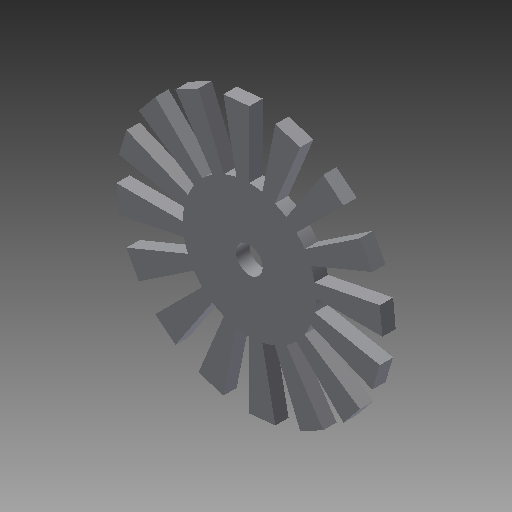
# Autodesk Inventor part: encoder
Saved by Autodesk Inventor 2017 (Build 210142000, 142)
## iProperties
Created: 2016-09-12
Part Number: encoder
Material: Generic
Document SubType Name: Modeling
Designer: Paulo Loma
Density: 1 g/cm^3
Appearance: Default
Author: Paulo Loma
Autodesk Inventor part; units mm, degrees
ref_plane "YZ Plane" through (0, 0, 0) normal (1, 0, 0) x (0, 1, 0)
ref_plane "XZ Plane" through (0, 0, 0) normal (0, 1, 0) x (-1, 0, 0)
ref_plane "XY Plane" through (0, 0, 0) normal (0, 0, 1) x (1, 0, 0)
sketch "Sketch1" plane through (0, 0, 0) normal (0, 0, 1) x (1, 0, 0)
  circle A0 centre (0, 0) radius 1
  circle A1 centre (0, 0) radius 5
  line L0 (1.9509, 9.8079) -> (3.8268, 9.2388)
  line L1 (5.5557, 8.3147) -> (7.0711, 7.0711)
  line L2 (8.3147, 5.5557) -> (9.2388, 3.8268)
  line L3 (9.8079, 1.9509) -> (10, 0)
  line L4 (9.8079, -1.9509) -> (9.2388, -3.8268)
  line L5 (8.3147, -5.5557) -> (7.0711, -7.0711)
  line L6 (5.5557, -8.3147) -> (3.8268, -9.2388)
  line L7 (1.9509, -9.8079) -> (0, -10)
  line L8 (-1.9509, -9.8079) -> (-3.8268, -9.2388)
  line L9 (-5.5557, -8.3147) -> (-7.0711, -7.0711)
  line L10 (-8.3147, -5.5557) -> (-9.2388, -3.8268)
  line L11 (-9.8079, -1.9509) -> (-10, 0)
  line L12 (-9.8079, 1.9509) -> (-9.2388, 3.8268)
  line L13 (-8.3147, 5.5557) -> (-7.0711, 7.0711)
  line L14 (-5.5557, 8.3147) -> (-3.8268, 9.2388)
  line L15 (-1.9509, 9.8079) -> (0, 10)
  line L16 (-3.8268, 9.2388) -> (-1.9134, 4.6194)
  line L17 (-5.5557, 8.3147) -> (-2.7779, 4.1573)
  line L18 (-9.2388, -3.8268) -> (-4.6194, -1.9134)
  line L19 (-8.3147, -5.5557) -> (-4.1573, -2.7779)
  line L20 (-7.0711, -7.0711) -> (-3.5355, -3.5355)
  line L21 (-5.5557, -8.3147) -> (-2.7779, -4.1573)
  line L22 (-1.9509, -9.8079) -> (-0.9755, -4.9039)
  line L23 (-3.8268, -9.2388) -> (-1.9134, -4.6194)
  line L24 (0, -5) -> (0, -10)
  line L25 (0.9755, -4.9039) -> (1.9509, -9.8079)
  line L26 (-0.3827, 0.9239) -> (0.3827, -0.9239)
  line L27 (1.9134, -4.6194) -> (3.8268, -9.2388)
  line L28 (-0.5556, 0.8315) -> (0.5556, -0.8315)
  line L29 (2.7779, -4.1573) -> (5.5557, -8.3147)
  line L30 (3.5355, -3.5355) -> (7.0711, -7.0711)
  line L31 (4.1573, -2.7779) -> (8.3147, -5.5557)
  line L32 (4.6194, -1.9134) -> (9.2388, -3.8268)
  line L33 (4.9039, -0.9755) -> (9.8079, -1.9509)
  line L34 (5, 0) -> (10, 0)
  line L35 (4.9039, 0.9755) -> (9.8079, 1.9509)
  line L36 (-0.9239, -0.3827) -> (0.9239, 0.3827)
  line L37 (4.6194, 1.9134) -> (9.2388, 3.8268)
  line L38 (-0.8315, -0.5556) -> (0.8315, 0.5556)
  line L39 (4.1573, 2.7779) -> (8.3147, 5.5557)
  line L40 (-0.7071, -0.7071) -> (0.7071, 0.7071)
  line L41 (3.5355, 3.5355) -> (7.0711, 7.0711)
  line L42 (-0.5556, -0.8315) -> (0.5556, 0.8315)
  line L43 (2.7779, 4.1573) -> (5.5557, 8.3147)
  line L44 (-0.3827, -0.9239) -> (0.3827, 0.9239)
  line L45 (1.9134, 4.6194) -> (3.8268, 9.2388)
  line L46 (-0.1951, -0.9808) -> (0.1951, 0.9808)
  line L47 (0.9755, 4.9039) -> (1.9509, 9.8079)
  line L48 (0, 10) -> (0, 5)
  line L49 (0, 1) -> (0, -1)
  line L50 (-1.9509, 9.8079) -> (-0.9755, 4.9039)
  line L51 (-0.1951, 0.9808) -> (0.1951, -0.9808)
  line L52 (-7.0711, 7.0711) -> (-3.5355, 3.5355)
  line L53 (-0.7071, 0.7071) -> (0.7071, -0.7071)
  line L54 (-8.3147, 5.5557) -> (-4.1573, 2.7779)
  line L55 (-0.8315, 0.5556) -> (0.8315, -0.5556)
  line L56 (-9.2388, 3.8268) -> (-4.6194, 1.9134)
  line L57 (-0.9239, 0.3827) -> (0.9239, -0.3827)
  line L58 (-0.9808, 0.1951) -> (0.9808, -0.1951)
  line L59 (-10, 0) -> (-5, 0)
  line L60 (-1, 0) -> (1, 0)
  line L61 (-9.8079, -1.9509) -> (-4.9039, -0.9755)
  line L62 (-0.9808, -0.1951) -> (0.9808, 0.1951)
  line L63 (-9.8079, 1.9509) -> (-4.9039, 0.9755)
  line L64 (-0.9808, 0.1951) -> (0, 0)
  dimension "d1" = 2
  constraints: 130 end point, 60 perpendicular, 3 vertical, 2 coincident, 2 midpoint, 101 other
extrude "Extrusion2" add sketch "Sketch1" along normal blind 1
body "Solid2"
